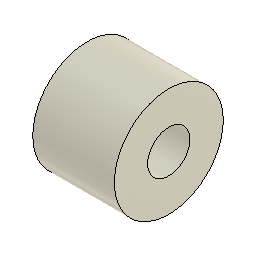
0.5 OD Spacer, 0.375 (Nylon) v2 (Autodesk Fusion 360 design; units mm, degrees)
Autodesk Fusion 360 part; units mm, degrees
sketch "sketch 176" plane through (0, 0, 0) normal (1, 0, 0) x (0, 1, 0)
  circle A0 centre (0, 0) radius 6.35
  circle A1 centre (0, 0) radius 2.4638
extrude "Extrude1" add sketch "sketch 176" along normal blind 9.525
